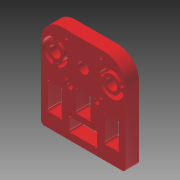
# Autodesk Inventor part: gantry3
Saved by Autodesk Inventor 2012 SP1 (Build 160190100, 190)
## iProperties
Created: 2011-10-14
Part Number: gantry3
Document SubType Name: Modeling
Designer: cramera
Density: 0.952 g/cm^3
Material: High Density Polyethylene
Mass: 48.2645 g
Surface Area: 212.552 cm^2
Volume: 50.698 cm^3
Autodesk Inventor part; units mm, degrees
ref_plane "YZ Plane" through (0, 0, 0) normal (1, 0, 0) x (0, 1, 0)
ref_plane "XZ Plane" through (0, 0, 0) normal (0, 1, 0) x (-1, 0, 0)
ref_plane "XY Plane" through (0, 0, 0) normal (0, 0, 1) x (1, 0, 0)
derived "skeleton.ipt"
sketch "DRILL-THROUGH" plane through (0, 0, 0) normal (0, 0, 1) x (1, 0, 0)
  arc A0 (722.0241, 509.6155) -> (720.4366, 511.203) centre (720.4366, 509.6155) ccw
  arc A1 (687.8611, 509.6155) -> (689.4486, 508.028) centre (689.4486, 509.6155) ccw
  arc A2 (691.0361, 478.6275) -> (689.4486, 480.215) centre (689.4486, 478.6275) ccw
  arc A3 (689.4486, 480.215) -> (687.8611, 478.6275) centre (689.4486, 478.6275) ccw
  arc A4 (720.4366, 508.028) -> (722.0241, 509.6155) centre (720.4366, 509.6155) ccw
  arc A5 (689.4486, 511.203) -> (687.8611, 509.6155) centre (689.4486, 509.6155) ccw
  arc A6 (720.4366, 511.203) -> (718.8491, 509.6155) centre (720.4366, 509.6155) ccw
  arc A7 (687.8611, 478.6275) -> (689.4486, 477.04) centre (689.4486, 478.6275) ccw
  arc A8 (689.4486, 477.04) -> (691.0361, 478.6275) centre (689.4486, 478.6275) ccw
  arc A9 (720.4366, 480.215) -> (718.8491, 478.6275) centre (720.4366, 478.6275) ccw
  arc A10 (722.0241, 478.6275) -> (720.4366, 480.215) centre (720.4366, 478.6275) ccw
  arc A11 (720.4366, 477.04) -> (722.0241, 478.6275) centre (720.4366, 478.6275) ccw
  arc A12 (718.8491, 478.6275) -> (720.4366, 477.04) centre (720.4366, 478.6275) ccw
  arc A13 (718.8491, 509.6155) -> (720.4366, 508.028) centre (720.4366, 509.6155) ccw
  arc A14 (691.0361, 509.6155) -> (689.4486, 511.203) centre (689.4486, 509.6155) ccw
  arc A15 (689.4486, 508.028) -> (691.0361, 509.6155) centre (689.4486, 509.6155) ccw
  constraints: 32 point on circle, 16 centre point
sketch "POCKET_1-4" plane through (0, 0, 0) normal (0, 0, 1) x (1, 0, 0)
  arc A0 (704.9426, 481.4215) -> (717.6426, 494.1215) centre (704.9426, 494.1215) ccw
  arc A1 (717.6426, 494.1215) -> (704.9426, 506.8215) centre (704.9426, 494.1215) ccw
  arc A2 (704.9426, 506.8215) -> (692.2426, 494.1215) centre (704.9426, 494.1215) ccw
  arc A3 (692.2426, 494.1215) -> (704.9426, 481.4215) centre (704.9426, 494.1215) ccw
  constraints: 8 point on circle, 4 centre point
sketch "POCKET_1-8" plane through (0, 0, 0) normal (0, 0, 1) x (1, 0, 0)
  arc A0 (716.6266, 509.6155) -> (720.4366, 505.8055) centre (720.4366, 509.6155) ccw
  arc A1 (720.4366, 505.8055) -> (724.2466, 509.6155) centre (720.4366, 509.6155) ccw
  arc A2 (685.6386, 478.6275) -> (689.4486, 474.8175) centre (689.4486, 478.6275) ccw
  arc A3 (720.4366, 513.4255) -> (716.6266, 509.6155) centre (720.4366, 509.6155) ccw
  arc A4 (724.2466, 478.6275) -> (720.4366, 482.4375) centre (720.4366, 478.6275) ccw
  arc A5 (689.4486, 513.4255) -> (685.6386, 509.6155) centre (689.4486, 509.6155) ccw
  arc A6 (693.2586, 509.6155) -> (689.4486, 513.4255) centre (689.4486, 509.6155) ccw
  arc A7 (724.2466, 509.6155) -> (720.4366, 513.4255) centre (720.4366, 509.6155) ccw
  arc A8 (689.4486, 505.8055) -> (693.2586, 509.6155) centre (689.4486, 509.6155) ccw
  arc A9 (716.6266, 478.6275) -> (720.4366, 474.8175) centre (720.4366, 478.6275) ccw
  arc A10 (720.4366, 474.8175) -> (724.2466, 478.6275) centre (720.4366, 478.6275) ccw
  arc A11 (720.4366, 482.4375) -> (716.6266, 478.6275) centre (720.4366, 478.6275) ccw
  arc A12 (685.6386, 509.6155) -> (689.4486, 505.8055) centre (689.4486, 509.6155) ccw
  arc A13 (689.4486, 482.4375) -> (685.6386, 478.6275) centre (689.4486, 478.6275) ccw
  arc A14 (693.2586, 478.6275) -> (689.4486, 482.4375) centre (689.4486, 478.6275) ccw
  arc A15 (689.4486, 474.8175) -> (693.2586, 478.6275) centre (689.4486, 478.6275) ccw
  constraints: 32 point on circle, 16 centre point
sketch "STOCK_12MM" plane through (0, 0, 0) normal (0, 0, 1) x (1, 0, 0)
  line L0 (457.2, 0) -> (914.4, 0)
  line L1 (914.4, 0) -> (914.4, 914.4)
  line L2 (914.4, 914.4) -> (457.2, 914.4)
  line L3 (457.2, 914.4) -> (457.2, 0)
  line L4 (0, 0) -> (457.2, 0)
  line L5 (457.2, 0) -> (457.2, 914.4)
  line L6 (457.2, 914.4) -> (0, 914.4)
  line L7 (0, 914.4) -> (0, 0)
  constraints: 16 end point
sketch "THROUGH-CUT" plane through (0, 0, 0) normal (0, 0, 1) x (1, 0, 0)
  arc A0 (701.0281, 475.0715) -> (698.7831, 472.8264) centre (699.9056, 473.949) ccw
  arc A1 (692.7506, 440.2948) -> (694.9956, 438.0497) centre (693.8731, 439.1722) ccw
  line L0 (694.9956, 438.0497) -> (714.8895, 438.0497)
  arc A2 (714.8895, 438.0497) -> (717.1346, 440.2948) centre (716.012, 439.1722) ccw
  line L1 (717.1346, 440.2948) -> (717.1346, 448.1237)
  arc A3 (717.1346, 448.1237) -> (714.8895, 450.3687) centre (716.012, 449.2462) ccw
  line L2 (714.8895, 450.3687) -> (694.9956, 450.3687)
  arc A4 (694.9956, 450.3687) -> (692.7506, 448.1237) centre (693.8731, 449.2462) ccw
  line L3 (692.7506, 448.1237) -> (692.7506, 440.2948)
  arc A5 (673.1926, 446.8683) -> (673.1926, 444.6232) centre (674.3151, 445.7458) ccw
  arc A6 (673.1926, 444.6232) -> (675.4376, 444.6232) centre (674.3151, 445.7458) ccw
  line L4 (675.4376, 444.6232) -> (683.2665, 444.6232)
  arc A7 (683.2665, 444.6232) -> (685.5116, 446.8683) centre (684.389, 445.7458) ccw
  line L5 (685.5116, 446.8683) -> (685.5116, 466.7622)
  arc A8 (685.5116, 466.7622) -> (683.2665, 469.0072) centre (684.389, 467.8847) ccw
  line L6 (683.2665, 469.0072) -> (675.4376, 469.0072)
  arc A9 (675.4376, 469.0072) -> (673.1926, 469.0072) centre (674.3151, 467.8847) ccw
  arc A10 (673.1926, 469.0072) -> (673.1926, 466.7622) centre (674.3151, 467.8847) ccw
  line L7 (673.1926, 466.7622) -> (673.1926, 446.8683)
  circle A11 centre (679.5426, 494.1215) radius 5
  arc A12 (666.8426, 434.8747) -> (670.0176, 431.6997) centre (670.0176, 434.8747) ccw
  line L8 (670.0176, 431.6997) -> (739.8676, 431.6997)
  arc A13 (700.1801, 494.1215) -> (704.9426, 489.359) centre (704.9426, 494.1215) ccw
  line L9 (743.0426, 434.8747) -> (743.0426, 497.2965)
  arc A14 (743.0426, 497.2965) -> (723.9926, 516.3465) centre (723.9926, 497.2965) ccw
  line L10 (723.9926, 516.3465) -> (685.8926, 516.3465)
  arc A15 (685.8926, 516.3465) -> (666.8426, 497.2965) centre (685.8926, 497.2965) ccw
  line L11 (666.8426, 497.2965) -> (666.8426, 434.8747)
  arc A16 (724.3736, 446.8683) -> (726.6186, 444.6232) centre (725.4961, 445.7458) ccw
  line L12 (726.6186, 444.6232) -> (734.4475, 444.6232)
  arc A17 (734.4475, 444.6232) -> (736.6926, 446.8683) centre (735.57, 445.7458) ccw
  line L13 (736.6926, 446.8683) -> (736.6926, 466.7622)
  arc A18 (736.6926, 466.7622) -> (734.4475, 469.0072) centre (735.57, 467.8847) ccw
  line L14 (734.4475, 469.0072) -> (726.6186, 469.0072)
  arc A19 (726.6186, 469.0072) -> (724.3736, 466.7622) centre (725.4961, 467.8847) ccw
  line L15 (724.3736, 466.7622) -> (724.3736, 446.8683)
  arc A20 (692.9411, 476.2777) -> (690.5281, 473.8647) centre (692.9411, 473.8647) ccw
  arc A21 (690.5281, 473.8647) -> (692.9411, 471.4517) centre (692.9411, 473.8647) ccw
  arc A22 (739.8676, 431.6997) -> (743.0426, 434.8747) centre (739.8676, 434.8747) ccw
  arc A23 (692.9411, 471.4517) -> (695.3541, 473.8647) centre (692.9411, 473.8647) ccw
  arc A24 (695.3541, 473.8647) -> (692.9411, 476.2777) centre (692.9411, 473.8647) ccw
  arc A25 (704.9426, 489.359) -> (709.7051, 494.1215) centre (704.9426, 494.1215) ccw
  arc A26 (709.7051, 494.1215) -> (704.9426, 498.884) centre (704.9426, 494.1215) ccw
  arc A27 (704.9426, 498.884) -> (700.1801, 494.1215) centre (704.9426, 494.1215) ccw
  arc A28 (716.9441, 476.2777) -> (714.5311, 473.8647) centre (716.9441, 473.8647) ccw
  arc A29 (714.5311, 473.8647) -> (716.9441, 471.4517) centre (716.9441, 473.8647) ccw
  arc A30 (716.9441, 471.4517) -> (719.3571, 473.8647) centre (716.9441, 473.8647) ccw
  arc A31 (719.3571, 473.8647) -> (716.9441, 476.2777) centre (716.9441, 473.8647) ccw
  circle A32 centre (730.3426, 494.1215) radius 5
  line L16 (698.7831, 472.8264) -> (698.7831, 458.0126)
  arc A33 (698.7831, 458.0126) -> (701.0281, 455.7675) centre (699.9056, 456.89) ccw
  line L17 (701.0281, 455.7675) -> (708.857, 455.7675)
  arc A34 (708.857, 455.7675) -> (711.1021, 458.0126) centre (709.9795, 456.89) ccw
  line L18 (711.1021, 458.0126) -> (711.1021, 472.8264)
  arc A35 (711.1021, 472.8264) -> (708.857, 475.0715) centre (709.9795, 473.949) ccw
  line L19 (708.857, 475.0715) -> (701.0281, 475.0715)
  arc A36 (681.2698, 485.1377) -> (683.4068, 483.6483) centre (682.8573, 485.1377) ccw
  arc A37 (683.4068, 483.6483) -> (683.4068, 504.5946) centre (679.5426, 494.1215) ccw
  arc A38 (683.4068, 504.5946) -> (681.2698, 503.1053) centre (682.8573, 503.1053) ccw
  line L20 (681.2698, 503.1053) -> (681.2698, 502.9969)
  arc A39 (681.2698, 502.9969) -> (682.3018, 501.5097) centre (682.8573, 502.9969) ccw
  arc A40 (682.3018, 486.7332) -> (682.3018, 501.5097) centre (679.5426, 494.1215) ccw
  arc A41 (682.3018, 486.7332) -> (681.2698, 485.2461) centre (682.8573, 485.2461) ccw
  line L21 (681.2698, 485.2461) -> (681.2698, 485.1377)
  arc A42 (740.8157, 490.2573) -> (739.3264, 492.3943) centre (739.3264, 490.8068) ccw
  line L22 (739.3264, 492.3943) -> (739.218, 492.3943)
  arc A43 (739.218, 492.3943) -> (737.7308, 491.3622) centre (739.218, 490.8068) ccw
  arc A44 (722.9543, 491.3622) -> (737.7308, 491.3622) centre (730.3426, 494.1215) ccw
  arc A45 (722.9543, 491.3622) -> (721.4671, 492.3943) centre (721.4671, 490.8068) ccw
  line L23 (721.4671, 492.3943) -> (721.3588, 492.3943)
  arc A46 (721.3588, 492.3943) -> (719.8694, 490.2573) centre (721.3588, 490.8068) ccw
  arc A47 (719.8694, 490.2573) -> (740.8157, 490.2573) centre (730.3426, 494.1215) ccw
  arc A48 (675.6783, 483.6483) -> (677.8154, 485.1377) centre (676.2279, 485.1377) ccw
  arc A49 (675.6783, 504.5946) -> (675.6783, 483.6483) centre (679.5426, 494.1215) ccw
  arc A50 (677.8154, 503.1053) -> (675.6783, 504.5946) centre (676.2279, 503.1053) ccw
  line L24 (677.8154, 503.1053) -> (677.8154, 502.9969)
  arc A51 (676.7833, 501.5097) -> (677.8154, 502.9969) centre (676.2279, 502.9969) ccw
  arc A52 (676.7833, 501.5097) -> (676.7833, 486.7332) centre (679.5426, 494.1215) ccw
  arc A53 (677.8154, 485.2461) -> (676.7833, 486.7332) centre (676.2279, 485.2461) ccw
  line L25 (677.8154, 485.2461) -> (677.8154, 485.1377)
  arc A54 (719.8694, 497.9857) -> (721.3588, 495.8487) centre (721.3588, 497.4362) ccw
  arc A55 (740.8157, 497.9857) -> (719.8694, 497.9857) centre (730.3426, 494.1215) ccw
  arc A56 (739.3264, 495.8487) -> (740.8157, 497.9857) centre (739.3264, 497.4362) ccw
  line L26 (739.3264, 495.8487) -> (739.218, 495.8487)
  arc A57 (737.7308, 496.8808) -> (739.218, 495.8487) centre (739.218, 497.4362) ccw
  arc A58 (737.7308, 496.8808) -> (722.9543, 496.8808) centre (730.3426, 494.1215) ccw
  arc A59 (721.4671, 495.8487) -> (722.9543, 496.8808) centre (721.4671, 497.4362) ccw
  line L27 (721.4671, 495.8487) -> (721.3588, 495.8487)
  dimension "d9" = 10
  dimension "d10" = 10
  constraints: 116 point on circle, 60 centre point, 56 end point
  measures "d9" diameter of A11
  measures "d10" diameter of A32
extrude "Extrusion1" add sketch "THROUGH-CUT" along normal blind 12
extrude "Extrusion2" cut sketch "POCKET_1-8" along normal blind 3.175
extrude "Extrusion3" cut sketch "POCKET_1-4" along normal blind 6.35
extrude "Extrusion4" cut sketch "DRILL-THROUGH" along normal through all
equation "\"d10\" = d9"
equation "\"d1\" = StockThickness"
equation "\"StockThickness\" = 12"
body "Solid1"
